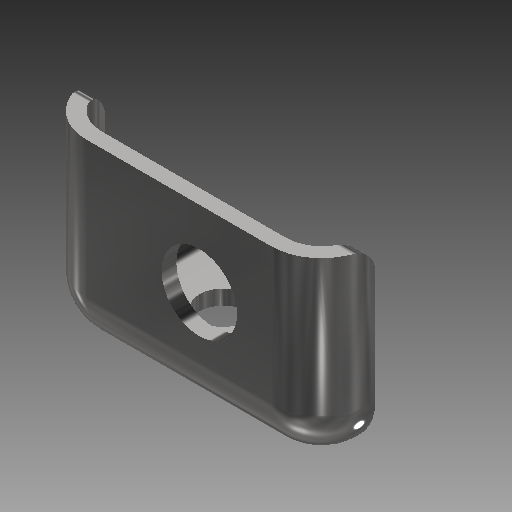
# Autodesk Inventor part: 314-08
Saved by Autodesk Inventor 2019 (Build 230136000, 136)
## iProperties
Company: Autodesk Inc.
Created: 2007-10-25
Part Number: 314-08
Document SubType Name: Modeling
Designer: Autodesk Inc.
Density: 7.85 g/cm^3
Mass: 44.104 g
Surface Area: 50.9446 cm^2
Volume: 5.61835 cm^3
Material: Steel
Description: FRONT CORNER BRACKET - R
Appearance: Steel - Polished
Component Category: Lower Component
Author: Inventor
Autodesk Inventor part; units mm, degrees
ref_plane "YZ Plane" through (0, 0, 0) normal (1, 0, 0) x (0, 1, 0)
ref_plane "XZ Plane" through (0, 0, 0) normal (0, 1, 0) x (-1, 0, 0)
ref_plane "XY Plane" through (0, 0, 0) normal (0, 0, 1) x (1, 0, 0)
sketch "Sketch1" plane through (0, 0, 0) normal (0, 0, 1) x (1, 0, 0)
  line L0 (-24.1415, 15.787) -> (24.1415, 15.787)
  line L1 (24.1415, 15.787) -> (24.1415, -15.787)
  line L2 (24.1415, -15.787) -> (-24.1415, -15.787)
  line L3 (-24.1415, -15.787) -> (-24.1415, 15.787)
  point P0 (0, 0)
  dimension "d0" = 31.574
  dimension "d1" = 48.283
  dimension "d2" = 24.1415
  dimension "d3" = 15.787
  constraints: 8 end point, 2 parallel, 1 horizontal, 1 perpendicular
  measures "d0" distance of L2.end L0.start
  measures "d1" distance of L0.start L0.end
  measures "d2" distance from line of point (0, 0) L3
  measures "d3" distance from line of point (0, 0) L0
extrude "Extrusion1" add sketch "Sketch1" against normal blind 26.136
fillet "Fillet1" radius 8.5 5 edges at (0, -15.787, 0) (24.1415, 0, 0) (-24.1415, 0, 0) (-24.1415, -15.787, -13.068) (24.1415, -15.787, -13.068)
shell "Shell1" thickness 2.5 removed faces 2 at (5.2138, 15.787, -17.424) at (-5.2138, 5.2623, -26.136)
sketch "Sketch2" plane through (-24.1415, -7.287, -8.5) normal (-1, 0, 0) x (0, 0, 1)
  line L0 (0, 23.074) -> (-17.636, 23.074) projected
  line L1 (-17.636, 23.074) -> (-17.636, 0) projected
  line L2 (-17.636, -0.926) -> (-0.636, -0.926)
  line L3 (-0.636, -0.926) -> (-0.636, 23.074)
  line L4 (-0.636, 23.074) -> (-17.636, 23.074)
  line L5 (-17.636, 23.074) -> (-17.636, -0.926)
  point P0 (8.5, 7.287)
  dimension "d8" = 17
  dimension "d9" = 24
  constraints: 8 end point, 2 parallel, 2 point on line, 1 horizontal, 1 perpendicular
  measures "d8" distance of L2.start L2.end
  measures "d9" distance from line of L2 L0.start
extrude "Extrusion2" cut sketch "Sketch2" against normal through all
sketch "Sketch3" plane through (-15.6415, 15.787, 0) normal (0, 1, 0) x (1, 0, 0)
  line L0 (39.783, 8.5) -> (39.783, 9.136) projected
  line L1 (39.783, 9.136) -> (34.783, 9.136)
  line L2 (34.783, 9.136) -> (14.783, 26.136)
  line L3 (0, 26.136) -> (31.283, 26.136) projected
  line L4 (39.783, 9.136) -> (39.783, 26.136)
  line L5 (39.783, 26.136) -> (14.783, 26.136)
  point P0 (15.6415, 0)
  dimension "d12" = 5
  dimension "d13" = 20
  constraints: 8 end point, 2 perpendicular, 2 point on line, 1 collinear
  measures "d12" distance of L0.end L1.end
  measures "d13" horizontal distance of L2.end L1.end
extrude "Extrusion3" cut sketch "Sketch3" against normal through all
fillet "Fillet2" radius 4 6 edges at (-22.8303, -8.213, -26.136) (19.1415, -13.5967, -9.136) (-22.8303, -8.213, -9.136) (-22.8915, 15.787, -9.136) (22.8915, 15.787, -9.136) (-0.8585, -14.537, -26.136)
sketch "Sketch4" plane through (0, 0, 0) normal (0, 0, 1) x (1, 0, 0)
  line L0 (0.2618, -15.787) -> (-2.3288, -15.787) projected
  line L1 (0.2618, -15.787) -> (15.6415, -15.787) projected
  line L2 (-15.6415, -15.787) -> (15.6415, -15.787) projected
  line L3 (-15.6415, -15.787) -> (-2.3288, -15.787) projected
  line L4 (-24.1415, 11.787) -> (-24.1415, 13.9511) projected
  line L5 (-24.1415, 11.787) -> (-24.1415, -4.213) projected
  line L6 (-24.1415, -4.213) -> (-24.1415, -7.287) projected
  line L7 (-24.1415, 13.9511) -> (-24.1415, -7.287) projected
  point P0 (0, 0)
  point P1 (3.4645, 2.911)
  dimension "d17" = 27.606
  dimension "d18" = 18.698
  measures "d17" distance from line of point (3.464, 2.911) L7
  measures "d18" distance from line of L2 point (3.464, 2.911)
hole "Hole1" at (3.4645, 2.911, 0) direction (0, 0, -1) diameter 12.8 end through all
sketch "Sketch5" plane through (-15.6415, -15.787, -8.5) normal (0, -1, 0) x (1, 0, 0)
  line L0 (-8.5, -2.0766) -> (-8.5, -0.636) projected
  line L1 (12.706, 8.5) -> (25.506, 8.5) projected
  line L2 (0, 8.5) -> (31.283, 8.5) projected
  line L3 (31.283, 8.5) -> (0, 8.5) projected
  point P0 (15.6415, 8.5)
  point P1 (7.163, -7.48)
  dimension "d26" = 15.663
  dimension "d27" = 15.98
  measures "d26" distance from line of point (7.163, -7.48) L0
  measures "d27" distance from line of L2 point (7.163, -7.48)
hole "Hole2" at (-8.4785, -15.787, -15.98) direction (0, 1, 0) diameter 8 end through all
equation "\"d2\" = 0.5 * d1"
equation "\"d3\" = 0.5 * d0"
body "Solid1"
